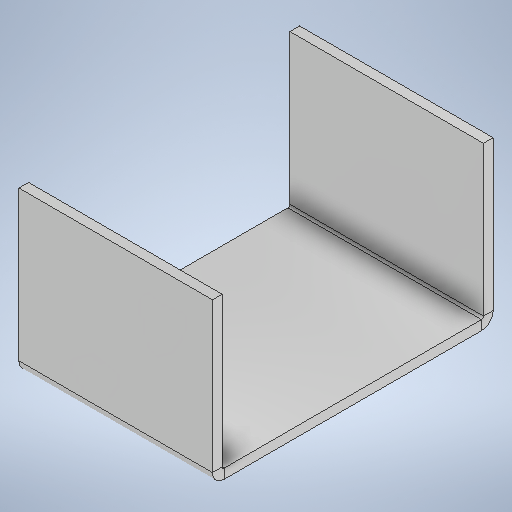
# Autodesk Inventor part: chanhui
Saved by Autodesk Inventor 2025.2 (Build 292293000, 293)
## iProperties
Created: 2025-03-25
Part Number: chanhui
Material: Aluminum 6061-AHC
Document SubType Name: Sheet Metal
Designer: chanh
Density: 2.7 g/cm^3
Sheet Metal Rule: Default_mm
Appearance: Aluminum - Dark
Author: chanh
Autodesk Inventor part; units mm, degrees
ref_plane "YZ Plane" through (0, 0, 0) normal (1, 0, 0) x (0, 1, 0)
ref_plane "XZ Plane" through (0, 0, 0) normal (0, 1, 0) x (-1, 0, 0)
ref_plane "XY Plane" through (0, 0, 0) normal (0, 0, 1) x (1, 0, 0)
sketch "Sketch1" plane through (0, 0, 0) normal (0, 1, 0) x (-1, 0, 0)
  line L0 (-15, 20.25) -> (15, 20.25)
  line L1 (15, 20.25) -> (15, -20.25)
  line L2 (15, -20.25) -> (-15, -20.25)
  line L3 (-15, -20.25) -> (-15, 20.25)
  line L4 (-15, 20.25) -> (15, -20.25) construction
  line L5 (15, 20.25) -> (-15, -20.25) construction
  point P0 (0, 0)
  dimension "d0" = 30
  dimension "d1" = 40.5
  measures "d0" distance of L1.end L2.end
  measures "d1" distance of L0.end L1.end
extrude "Plate1" add sketch "Sketch1" along normal blind 1.5
sketch "Sketch2" plane through (-15, 0, -21.75) normal (0, 0, 1) x (1, 0, 0)
  line L0 (30, 0) -> (0, 0)
  line L1 (0, 0) -> (0, 25)
  line L2 (0, 25) -> (30, 25)
  line L3 (30, 25) -> (30, 0)
  constraints: 8 end point
edge flange "Flange1" height 25 angle 90 thickness 1.5 bend radius 0.31 thickness toward (0, 0, 1) relief tear relief width 1.5 relief depth 0.75 corner gap 0.31 corner form 0 edges at (0, 1.5, -20.25) (0, 1.5, 20.25) wall of the first edge with corners at (15, 0, -21.75) (-15, 0, -21.75) (-15, 25, -21.75) (15, 25, -21.75)
bend "Bend1"
corner "Corner1"
equation "\"d2\" = Thickness"
equation "\"d3\" = BendReliefWidth"
equation "\"d4\" = BendReliefDepth"
equation "\"d5\" = MinimumRemnant"
equation "\"d6\" = TransitionRadius"
equation "\"d9\" = BendRadius"
equation "\"d10\" = CornerReliefSize"
equation "\"d11\" = GapSize"
equation "\"d12\" = JacobiRadiusSize"
equation "\"BendReliefWidth\" = Thickness"
equation "\"BendReliefDepth\" = 0.5 * Thickness"
equation "\"CornerReliefSize\" = 4 * Thickness"
equation "\"MinimumRemnant\" = 2 * Thickness"
equation "\"TransitionRadius\" = BendRadius"
equation "\"JacobiRadiusSize\" = BendRadius"
equation "\"GapSize\" = Thickness"
equation "\"Thickness\" = 1.5"
equation "\"BendRadius\" = 0.31"
body "Solid1"
